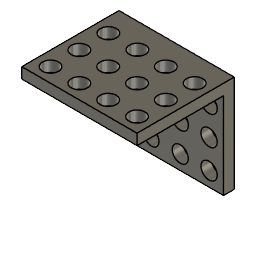
Perfil3x4 (Autodesk Fusion 360 design; units mm, degrees)
Autodesk Fusion 360 part; units mm, degrees
sketch "Boceto1" plane through (0, 0, 0) normal (0, 0, 1) x (1, 0, 0)
  line L0 (0, 0) -> (-31.9991, 0)
  line L1 (-31.9991, 0) -> (-31.9991, 24)
  line L2 (0, 24) -> (0, 0)
  circle A0 centre (-4, 20) radius 2.2361
  circle A1 centre (-4, 12) radius 2.2361
  circle A2 centre (-4, 4) radius 2.2361
  line L3 (-4, 20) -> (-4, 12) construction
  line L4 (-4, 12) -> (-4, 4) construction
  circle A3 centre (-12, 20) radius 2.2361
  line L5 (-4, 20) -> (-12, 20) construction
  circle A4 centre (-19.9992, 20.1116) radius 2.2361
  line L6 (-12, 20) -> (-19.9992, 20.1116) construction
  circle A5 centre (-12, 12) radius 2.2361
  circle A6 centre (-20, 12) radius 2.2361
  circle A7 centre (-12, 4) radius 2.2361
  circle A8 centre (-20, 4) radius 2.2361
  circle A9 centre (-27.9991, 20.0598) radius 2.2361
  line L7 (-19.9992, 20.1116) -> (-27.9991, 20.0598) construction
  circle A10 centre (-28, 12) radius 2.2361
  circle A11 centre (-28, 4) radius 2.2361
  line L8 (0, 24) -> (0, 27)
  line L9 (0, 27) -> (-31.9991, 27)
  line L10 (-31.9991, 27) -> (-31.9991, 24)
  dimension "d1" = 24
  dimension "d2" = 4.4721
  dimension "d3" = 16
  dimension "d4" = 4
  dimension "d5" = 4
  dimension "d6" = 4
  dimension "d7" = 3
  constraint horizontal L0
  constraint vertical L1
  constraint vertical L2
  constraint coincident L0.start L2.end
  constraint coincident A0.centre L3.start
  constraint coincident A1.centre L3.end
  constraint vertical L3
  constraint coincident A2.centre L4.end
  constraint parallel L3 L4
  constraint equal L3 L4
  constraint equal A1 A2
  constraint equal A0 A1
  constraint coincident A3.centre L5.end
  constraint equal A0 A3
  constraint equal L3 L5
  constraint coincident A4.centre L6.end
  constraint equal L5 L6
  constraint equal A3 A4
  constraint equal A7 A8
  constraint equal A6 A7
  constraint equal A5 A6
  constraint equal A1 A5
  constraint coincident A9.centre L7.end
  constraint equal L6 L7
  constraint equal A10 A11
  constraint equal A9 A10
  constraint equal A4 A9
  constraint vertical L8
  constraint horizontal L9
  constraint vertical L10
  measures "d1" distance of L0.start L2.start
  measures "d2" diameter of A2
  measures "d3" distance of A0.centre A2.centre
  measures "d4" distance of L0 A2.centre
  measures "d5" distance of L2 L3
  measures "d6" distance of L1 A9.centre
  measures "d7" distance of L1.end L9.end
extrude "Extruir1" add sketch "Boceto1" along normal blind 3
sketch "Boceto2" plane through (0, 0, 0) normal (0, 0, -1) x (1, 0, 0)
  circle A0 centre (-19.9992, -20.1116) radius 2.2361
  circle A1 centre (-20, -12) radius 2.2361
  circle A2 centre (-28, -4) radius 2.2361
  circle A3 centre (-27.9991, -20.0598) radius 2.2361
  circle A4 centre (-12, -20) radius 2.2361
  circle A5 centre (-12, -4) radius 2.2361
  circle A6 centre (-20, -4) radius 2.2361
  circle A7 centre (-12, -12) radius 2.2361
  circle A8 centre (-28, -12) radius 2.2361
  circle A9 centre (-4, -12) radius 2.2361
  circle A10 centre (-4, -4) radius 2.2361
  circle A11 centre (-4, -20) radius 2.2361
  line L0 (0, -27) -> (0, 0)
  line L1 (0, 0) -> (-31.9991, 0)
  line L2 (-31.9991, 0) -> (-31.9991, -27)
  line L3 (-31.9991, -27) -> (0, -27)
  line L4 (0, -27) -> (-31.9991, -27)
  line L5 (-31.9991, -27) -> (-31.9991, -24)
  line L6 (-31.9991, -24) -> (0, -24)
  line L7 (0, -24) -> (0, -27)
  dimension "d10" = 3
  constraint horizontal L4
  constraint vertical L5
  constraint horizontal L6
  constraint vertical L7
  constraint coincident L2 L5.end
  constraint coincident L0.start L3.end
  measures "d10" distance of L0.start L6.end
extrude "Extruir2" add sketch "Boceto2" along normal blind 24 contours L0 L2 L3 L4 L5 L6 L7
sketch "Boceto3" plane through (0, 24, 0) normal (0, -1, 0) x (1, 0, 0)
  line L0 (0, 0) -> (-31.9991, 0)
  line L1 (-31.9991, 0) -> (-31.9991, -24)
  line L2 (-31.9991, -24) -> (0, -24)
  line L3 (0, -24) -> (0, 0)
  circle A0 centre (-27.9991, -20) radius 2.1
  circle A1 centre (-27.9991, -12) radius 2.1
  circle A2 centre (-27.9991, -4) radius 2.1
  line L4 (-27.9991, -4) -> (-27.9991, -12) construction
  line L5 (-27.9991, -12) -> (-27.9991, -20) construction
  line L6 (-27.9991, -20) -> (-27.9991, -24) construction
  circle A3 centre (-19.9991, -20) radius 2.1
  line L7 (-27.9991, -20) -> (-19.9991, -20) construction
  circle A4 centre (-3.9991, -20) radius 2.262
  circle A5 centre (-11.9991, -20) radius 2.2361
  line L8 (-3.9991, -20) -> (-11.9991, -20) construction
  line L9 (-11.9991, -20) -> (-19.9991, -20) construction
  circle A6 centre (-20, -12) radius 2.262
  circle A7 centre (-12, -12) radius 2.262
  circle A8 centre (-4, -12) radius 2.262
  circle A9 centre (-20, -4) radius 2.262
  circle A10 centre (-12, -4) radius 2.262
  circle A11 centre (-4, -4) radius 2.262
  dimension "d13" = 4.2
  dimension "d14" = 4
  dimension "d15" = 4
  dimension "d16" = 4
  dimension "d17" = 4
  dimension "d18" = 4
  dimension "d19" = 8
  constraint equal A1 A2
  constraint equal A0 A1
  constraint coincident A2.centre L4.start
  constraint coincident A1.centre L4.end
  constraint coincident A0.centre L5.end
  constraint equal L4 L5
  constraint parallel L5 L6
  constraint equal A0 A3
  constraint coincident A3.centre L7.end
  constraint equal L5 L7
  constraint coincident A4.centre L8.start
  constraint coincident A5.centre L8.end
  constraint equal L8 L9
  constraint equal L7 L8
  constraint equal A10 A11
  constraint equal A9 A10
  constraint equal A6 A9
  constraint equal A6 A7
  constraint equal A7 A8
  constraint equal A4 A8
  measures "d13" diameter of A0
  measures "d14" distance of L1 A0.centre
  measures "d15" distance of L1 A1.centre
  measures "d16" distance of L1 A2.centre
  measures "d17" distance of L0 A2.centre
  measures "d18" distance of A0.centre L6.end
  measures "d19" distance of A2.centre A1.centre
extrude "Extruir3" cut sketch "Boceto3" against normal blind 15 contours A0 | A1 | A2 | A3 | A4 | A5 | A6 | A7 | A8 | A9 | A10 | A11
